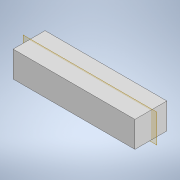
# Autodesk Inventor part: Battery
Saved by Autodesk Inventor 2021 (Build 250183000, 183)
## iProperties
Created: 2020-11-23
Part Number: Battery
Material: Generic
Document SubType Name: Modeling
Designer: Kanenas
Mass: 70 g
Surface Area: 39.54 cm^2
Volume: 12.688 cm^3
Density: 5.51702 g/cm^3
Appearance: Default
Author: Kanenas
Autodesk Inventor part; units mm, degrees
ref_plane "YZ Plane" through (0, 0, 0) normal (1, 0, 0) x (0, 1, 0)
ref_plane "XZ Plane" through (0, 0, 0) normal (0, 1, 0) x (-1, 0, 0)
sketch "Sketch1" plane through (0, 0, 0) normal (0, 1, 0) x (-1, 0, 0)
  line L0 (30.5, 8) -> (-30.5, 8)
  line L1 (-30.5, 8) -> (-30.5, -8)
  line L2 (-30.5, -8) -> (30.5, -8)
  line L3 (30.5, -8) -> (30.5, 8)
  line L4 (30.5, 8) -> (-30.5, -8) construction
  line L5 (-30.5, 8) -> (30.5, -8) construction
  point P0 (0, 0)
  dimension "d0" = 61
  dimension "d1" = 16
  constraints: 12 end point, 2 midpoint, 2 parallel, 1 horizontal, 1 perpendicular
  measures "d0" distance of L1.end L2.end
  measures "d1" distance of L2.end L0.start
extrude "Extrusion1" add sketch "Sketch1" along normal blind 13
body "Solid1"
